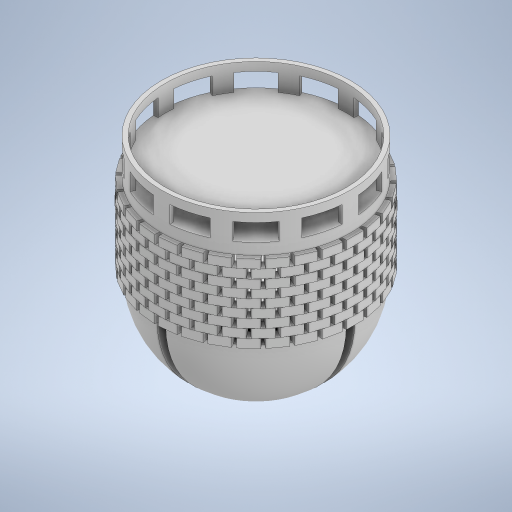
# Autodesk Inventor part: 背部建築 base
Saved by Autodesk Inventor 2024 (Build 280153000, 153)
## iProperties
Created: 2024-05-24
Part Number: 背部建築 base
Material: 一般
Document SubType Name: Modeling
Designer: User
Density: 1 g/cm^3
Appearance: 預設
Author: User
Autodesk Inventor part; units mm, degrees
(part 1 of 2)
ref_plane "YZ Plane" through (0, 0, 0) normal (1, 0, 0) x (0, 1, 0)
ref_plane "XZ Plane" through (0, 0, 0) normal (0, 1, 0) x (-1, 0, 0)
ref_plane "XY Plane" through (0, 0, 0) normal (0, 0, 1) x (1, 0, 0)
sketch "草圖1" plane through (0, 0, 0) normal (0, 1, 0) x (-1, 0, 0)
  circle A0 centre (0, 0) radius 11
  dimension "d0" = 22
  constraints: 1 centre point, 1 coincident
  measures "d0" diameter of A0
extrude "擠出1" add sketch "草圖1" along normal blind 1.3
sketch "草圖2" plane through (0, 1.3, 0) normal (0, 1, 0) x (1, 0, 0)
  line L0 (0, 0) -> (-10.9581, 0.9587)
  circle A0 centre (0, 0) radius 11 projected
  line L1 (0, 0) -> (-10.9581, -0.9587)
  line L2 (-13.6608, 0) -> (-12.5403, 0)
  circle A1 centre (0, 0) radius 10.5
  line L3 (0, 0) -> (-9.9694, -4.6488)
  line L4 (0, 0) -> (-9.0107, -6.3093)
  line L5 (0, 0) -> (-6.3093, -9.0107)
  line L6 (0, 0) -> (-4.6488, -9.9694)
  line L7 (0, 0) -> (-0.9587, -10.9581)
  line L8 (0, 0) -> (0.9587, -10.9581)
  line L9 (0, 0) -> (4.6488, -9.9694)
  line L10 (0, 0) -> (6.3093, -9.0107)
  line L11 (0, 0) -> (9.0107, -6.3093)
  line L12 (0, 0) -> (9.9694, -4.6488)
  line L13 (0, 0) -> (10.9581, -0.9587)
  line L14 (0, 0) -> (10.9581, 0.9587)
  line L15 (0, 0) -> (9.9694, 4.6488)
  line L16 (0, 0) -> (9.0107, 6.3093)
  line L17 (0, 0) -> (6.3093, 9.0107)
  line L18 (0, 0) -> (4.6488, 9.9694)
  line L19 (0, 0) -> (0.9587, 10.9581)
  line L20 (0, 0) -> (-0.9587, 10.9581)
  line L21 (0, 0) -> (-4.6488, 9.9694)
  line L22 (0, 0) -> (-6.3093, 9.0107)
  line L23 (0, 0) -> (-9.0107, 6.3093)
  line L24 (0, 0) -> (-9.9694, 4.6488)
  point P0 (9.5162, -4.4375)
  point P1 (8.6011, -6.0226)
  point P2 (10.46, 0.9151)
  point P3 (10.46, -0.9151)
  point P4 (8.6011, 6.0226)
  point P5 (9.5162, 4.4375)
  point P6 (4.4375, 9.5162)
  point P7 (6.0226, 8.6011)
  point P8 (-0.9151, 10.46)
  point P9 (0.9151, 10.46)
  point P10 (-6.0226, 8.6011)
  point P11 (-4.4375, 9.5162)
  point P12 (-9.5162, 4.4375)
  point P13 (-8.6011, 6.0226)
  point P14 (-10.46, -0.9151)
  point P15 (-10.46, 0.9151)
  point P16 (-8.6011, -6.0226)
  point P17 (-9.5162, -4.4375)
  point P18 (-4.4375, -9.5162)
  point P19 (-6.0226, -8.6011)
  point P20 (0.9151, -10.46)
  point P21 (-0.9151, -10.46)
  point P22 (6.0226, -8.6011)
  point P23 (4.4375, -9.5162)
  dimension "d5" = 21
  dimension "d3" = 5
  dimension "d4" = 5
  dimension "d8" = 360
  constraints: 50 end point, 2 horizontal, 1 coincident, 66 other
  measures "d3" angle of L2 L0
  measures "d4" angle of L2 L1
extrude "擠出2" add sketch "草圖2" along normal blind 2 contours A1 L1 A0 L0 | A1 L4 A0 L3 | A1 L6 A0 L5 | A1 L8 A0 L7 | A1 L10 A0 L9 | A1 L12 A0 L11 | A1 L14 A0 L13 | A1 L16 A0 L15 | A1 L18 A0 L17 | A1 L20 A0 L19 | A1 L22 A0 L21 | A1 L24 A0 L23
sketch "草圖3" plane through (0, 3.3, 0) normal (0, 1, 0) x (1, 0, 0)
  circle A0 centre (0, 0) radius 10.5
  circle A1 centre (0, 0) radius 11
  constraints: 2 centre point, 2 coincident
extrude "擠出3" add sketch "草圖3" along normal blind 1
sketch "草圖4" plane through (0, 0, 0) normal (0, -1, 0) x (1, 0, 0)
  circle A0 centre (0, 0) radius 11
  line L0 (-10.5, -1) -> (-11.5, -1)
  line L1 (-11.5, -1) -> (-11.5, 1)
  line L2 (-11.5, 1) -> (-10.5, 1)
  line L3 (-10.5, 1) -> (-10.5, -1)
  line L4 (-10.5, -1) -> (-11.5, 1) construction
  line L5 (-11.5, -1) -> (-10.5, 1) construction
  line L6 (-11.4566, -1.4128) -> (-10.4785, -1.2049)
  line L7 (-11.0408, -3.3691) -> (-11.4566, -1.4128)
  line L8 (-10.0626, -3.1612) -> (-11.0408, -3.3691)
  line L9 (-10.4785, -1.2049) -> (-10.0626, -3.1612)
  line L10 (-10.9125, -3.7639) -> (-9.999, -3.3572)
  line L11 (-10.099, -5.591) -> (-10.9125, -3.7639)
  line L12 (-9.1855, -5.1843) -> (-10.099, -5.591)
  line L13 (-9.999, -3.3572) -> (-9.1855, -5.1843)
  line L14 (-9.8915, -5.9505) -> (-9.0825, -5.3627)
  line L15 (-8.7159, -7.5685) -> (-9.8915, -5.9505)
  line L16 (-7.9069, -6.9808) -> (-8.7159, -7.5685)
  line L17 (-9.0825, -5.3627) -> (-7.9069, -6.9808)
  line L18 (-8.4381, -7.877) -> (-7.769, -7.1339)
  line L19 (-6.9519, -9.2153) -> (-8.4381, -7.877)
  line L20 (-6.2827, -8.4722) -> (-6.9519, -9.2153)
  line L21 (-7.769, -7.1339) -> (-6.2827, -8.4722)
  line L22 (-6.616, -9.4593) -> (-6.116, -8.5933)
  line L23 (-4.884, -10.4593) -> (-6.616, -9.4593)
  line L24 (-4.384, -9.5933) -> (-4.884, -10.4593)
  line L25 (-6.116, -8.5933) -> (-4.384, -9.5933)
  line L26 (-4.5048, -10.6281) -> (-4.1957, -9.6771)
  line L27 (-2.6026, -11.2462) -> (-4.5048, -10.6281)
  line L28 (-2.2936, -10.2951) -> (-2.6026, -11.2462)
  line L29 (-4.1957, -9.6771) -> (-2.2936, -10.2951)
  line L30 (-2.1966, -11.3325) -> (-2.0921, -10.338)
  line L31 (-0.2076, -11.5415) -> (-2.1966, -11.3325)
  line L32 (-0.103, -10.547) -> (-0.2076, -11.5415)
  line L33 (-2.0921, -10.338) -> (-0.103, -10.547)
  line L34 (0.2076, -11.5415) -> (0.103, -10.547)
  line L35 (2.1966, -11.3325) -> (0.2076, -11.5415)
  line L36 (2.0921, -10.338) -> (2.1966, -11.3325)
  line L37 (0.103, -10.547) -> (2.0921, -10.338)
  line L38 (2.6026, -11.2462) -> (2.2936, -10.2951)
  line L39 (4.5048, -10.6281) -> (2.6026, -11.2462)
  line L40 (4.1957, -9.6771) -> (4.5048, -10.6281)
  line L41 (2.2936, -10.2951) -> (4.1957, -9.6771)
  line L42 (4.884, -10.4593) -> (4.384, -9.5933)
  line L43 (6.616, -9.4593) -> (4.884, -10.4593)
  line L44 (6.116, -8.5933) -> (6.616, -9.4593)
  line L45 (4.384, -9.5933) -> (6.116, -8.5933)
  line L46 (6.9519, -9.2153) -> (6.2827, -8.4722)
  line L47 (8.4381, -7.877) -> (6.9519, -9.2153)
  line L48 (7.769, -7.1339) -> (8.4381, -7.877)
  line L49 (6.2827, -8.4722) -> (7.769, -7.1339)
  line L50 (8.7159, -7.5685) -> (7.9069, -6.9808)
  line L51 (9.8915, -5.9505) -> (8.7159, -7.5685)
  line L52 (9.0825, -5.3627) -> (9.8915, -5.9505)
  line L53 (7.9069, -6.9808) -> (9.0825, -5.3627)
  line L54 (10.099, -5.591) -> (9.1855, -5.1843)
  line L55 (10.9125, -3.7639) -> (10.099, -5.591)
  line L56 (9.999, -3.3572) -> (10.9125, -3.7639)
  line L57 (9.1855, -5.1843) -> (9.999, -3.3572)
  line L58 (11.0408, -3.3691) -> (10.0626, -3.1612)
  line L59 (11.4566, -1.4128) -> (11.0408, -3.3691)
  line L60 (10.4785, -1.2049) -> (11.4566, -1.4128)
  line L61 (10.0626, -3.1612) -> (10.4785, -1.2049)
  line L62 (11.5, -1) -> (10.5, -1)
  line L63 (11.5, 1) -> (11.5, -1)
  line L64 (10.5, 1) -> (11.5, 1)
  line L65 (10.5, -1) -> (10.5, 1)
  line L66 (11.4566, 1.4128) -> (10.4785, 1.2049)
  line L67 (11.0408, 3.3691) -> (11.4566, 1.4128)
  line L68 (10.0626, 3.1612) -> (11.0408, 3.3691)
  line L69 (10.4785, 1.2049) -> (10.0626, 3.1612)
  line L70 (10.9125, 3.7639) -> (9.999, 3.3572)
  line L71 (10.099, 5.591) -> (10.9125, 3.7639)
  line L72 (9.1855, 5.1843) -> (10.099, 5.591)
  line L73 (9.999, 3.3572) -> (9.1855, 5.1843)
  line L74 (9.8915, 5.9505) -> (9.0825, 5.3627)
  line L75 (8.7159, 7.5685) -> (9.8915, 5.9505)
  line L76 (7.9069, 6.9808) -> (8.7159, 7.5685)
  line L77 (9.0825, 5.3627) -> (7.9069, 6.9808)
  line L78 (8.4381, 7.877) -> (7.769, 7.1339)
  line L79 (6.9519, 9.2153) -> (8.4381, 7.877)
  line L80 (6.2827, 8.4722) -> (6.9519, 9.2153)
  line L81 (7.769, 7.1339) -> (6.2827, 8.4722)
  line L82 (6.616, 9.4593) -> (6.116, 8.5933)
  line L83 (4.884, 10.4593) -> (6.616, 9.4593)
  line L84 (4.384, 9.5933) -> (4.884, 10.4593)
  line L85 (6.116, 8.5933) -> (4.384, 9.5933)
  line L86 (4.5048, 10.6281) -> (4.1957, 9.6771)
  line L87 (2.6026, 11.2462) -> (4.5048, 10.6281)
  line L88 (2.2936, 10.2951) -> (2.6026, 11.2462)
  line L89 (4.1957, 9.6771) -> (2.2936, 10.2951)
  line L90 (2.1966, 11.3325) -> (2.0921, 10.338)
  line L91 (0.2076, 11.5415) -> (2.1966, 11.3325)
  line L92 (0.103, 10.547) -> (0.2076, 11.5415)
  line L93 (2.0921, 10.338) -> (0.103, 10.547)
  line L94 (-0.2076, 11.5415) -> (-0.103, 10.547)
  line L95 (-2.1966, 11.3325) -> (-0.2076, 11.5415)
  line L96 (-2.0921, 10.338) -> (-2.1966, 11.3325)
  line L97 (-0.103, 10.547) -> (-2.0921, 10.338)
  line L98 (-2.6026, 11.2462) -> (-2.2936, 10.2951)
  line L99 (-4.5048, 10.6281) -> (-2.6026, 11.2462)
  line L100 (-4.1957, 9.6771) -> (-4.5048, 10.6281)
  line L101 (-2.2936, 10.2951) -> (-4.1957, 9.6771)
  line L102 (-4.884, 10.4593) -> (-4.384, 9.5933)
  line L103 (-6.616, 9.4593) -> (-4.884, 10.4593)
  line L104 (-6.116, 8.5933) -> (-6.616, 9.4593)
  line L105 (-4.384, 9.5933) -> (-6.116, 8.5933)
  line L106 (-6.9519, 9.2153) -> (-6.2827, 8.4722)
  line L107 (-8.4381, 7.877) -> (-6.9519, 9.2153)
  line L108 (-7.769, 7.1339) -> (-8.4381, 7.877)
  line L109 (-6.2827, 8.4722) -> (-7.769, 7.1339)
  line L110 (-8.7159, 7.5685) -> (-7.9069, 6.9808)
  line L111 (-9.8915, 5.9505) -> (-8.7159, 7.5685)
  line L112 (-9.0825, 5.3627) -> (-9.8915, 5.9505)
  line L113 (-7.9069, 6.9808) -> (-9.0825, 5.3627)
  line L114 (-10.099, 5.591) -> (-9.1855, 5.1843)
  line L115 (-10.9125, 3.7639) -> (-10.099, 5.591)
  line L116 (-9.999, 3.3572) -> (-10.9125, 3.7639)
  line L117 (-9.1855, 5.1843) -> (-9.999, 3.3572)
  line L118 (-11.0408, 3.3691) -> (-10.0626, 3.1612)
  line L119 (-11.4566, 1.4128) -> (-11.0408, 3.3691)
  line L120 (-10.4785, 1.2049) -> (-11.4566, 1.4128)
  line L121 (-10.0626, 3.1612) -> (-10.4785, 1.2049)
  point P0 (-11, 0)
  dimension "d14" = 1
  dimension "d15" = 2
  dimension "d18" = 360
  constraints: 244 end point, 2 midpoint, 2 parallel, 1 coincident, 1 horizontal, 1 horizontal alignment, 1 perpendicular, 243 other
  measures "d14" distance of L1.end L2.end
  measures "d15" distance of L0.end L1.end
extrude "擠出4" add sketch "草圖4" along normal blind 1 contours A0 L62 L65 L64 | A0 L64 L63 L62 | L66 L69 L68 A0 | A0 L68 L67 L66 | L60 L59 L58 A0 | A0 L58 L61 L60 | L70 L73 L72 A0 | A0 L72 L71 L70 | L56 L55 L54 A0 | A0 L54 L57 L56 | L74 L77 L76 A0 | A0 L76 L75 L74 | L52 L51 L50 A0 | A0 L50 L53 L52 | L78 L81 L80 A0 | A0 L80 L79 L78 | L48 L47 L46 A0 | A0 L46 L49 L48 | L82 L85 L84 A0 | A0 L84 L83 L82 | L44 L43 L42 A0 | A0 L42 L45 L44 | L86 L89 L88 A0 | A0 L88 L87 L86 | L40 L39 L38 A0 | A0 L38 L41 L40 | L90 L93 L92 A0 | A0 L92 L91 L90 | L36 L35 L34 A0 | A0 L34 L37 L36 | L94 L97 L96 A0 | A0 L96 L95 L94 | L32 L31 L30 A0 | A0 L30 L33 L32 | L98 L101 L100 A0 | A0 L100 L99 L98 | L28 L27 L26 A0 | A0 L26 L29 L28 | L102 L105 L104 A0 | A0 L104 L103 L102 | L24 L23 L22 A0 | A0 L22 L25 L24 | L106 L109 L108 A0 | A0 L108 L107 L106 | L20 L19 L18 A0 | A0 L18 L21 L20 | L110 L113 L112 A0 | A0 L112 L111 L110 | L16 L15 L14 A0 | A0 L14 L17 L16 | L114 L117 L116 A0 | A0 L116 L115 L114 | L12 L11 L10 A0 | A0 L10 L13 L12 | L118 L121 L120 A0 | A0 L120 L119 L118 | L8 L7 L6 A0 | A0 L6 L9 L8 | L2 L3 L0 A0 | A0 L0 L1 L2
sketch "草圖5" plane through (0, -1, 0) normal (0, -1, 0) x (1, 0, 0)
  circle A0 centre (0, 0) radius 11
  line L0 (-1, 10.5) -> (1, 10.5)
  line L1 (1, 10.5) -> (1, 11.5)
  line L2 (1, 11.5) -> (-1, 11.5)
  line L3 (-1, 11.5) -> (-1, 10.5)
  line L4 (-1, 10.5) -> (1, 11.5) construction
  line L5 (1, 10.5) -> (-1, 11.5) construction
  line L6 (-1.2049, 10.4785) -> (-1.4128, 11.4566)
  line L7 (-1.4128, 11.4566) -> (-3.3691, 11.0408)
  line L8 (-3.1612, 10.0626) -> (-1.2049, 10.4785)
  line L9 (-3.3691, 11.0408) -> (-3.1612, 10.0626)
  line L10 (-3.3572, 9.999) -> (-3.7639, 10.9125)
  line L11 (-3.7639, 10.9125) -> (-5.591, 10.099)
  line L12 (-5.1843, 9.1855) -> (-3.3572, 9.999)
  line L13 (-5.591, 10.099) -> (-5.1843, 9.1855)
  line L14 (-5.3627, 9.0825) -> (-5.9505, 9.8915)
  line L15 (-5.9505, 9.8915) -> (-7.5685, 8.7159)
  line L16 (-6.9808, 7.9069) -> (-5.3627, 9.0825)
  line L17 (-7.5685, 8.7159) -> (-6.9808, 7.9069)
  line L18 (-7.1339, 7.769) -> (-7.877, 8.4381)
  line L19 (-7.877, 8.4381) -> (-9.2153, 6.9519)
  line L20 (-8.4722, 6.2827) -> (-7.1339, 7.769)
  line L21 (-9.2153, 6.9519) -> (-8.4722, 6.2827)
  line L22 (-8.5933, 6.116) -> (-9.4593, 6.616)
  line L23 (-9.4593, 6.616) -> (-10.4593, 4.884)
  line L24 (-9.5933, 4.384) -> (-8.5933, 6.116)
  line L25 (-10.4593, 4.884) -> (-9.5933, 4.384)
  line L26 (-9.6771, 4.1957) -> (-10.6281, 4.5048)
  line L27 (-10.6281, 4.5048) -> (-11.2462, 2.6026)
  line L28 (-10.2951, 2.2936) -> (-9.6771, 4.1957)
  line L29 (-11.2462, 2.6026) -> (-10.2951, 2.2936)
  line L30 (-10.338, 2.0921) -> (-11.3325, 2.1966)
  line L31 (-11.3325, 2.1966) -> (-11.5415, 0.2076)
  line L32 (-10.547, 0.103) -> (-10.338, 2.0921)
  line L33 (-11.5415, 0.2076) -> (-10.547, 0.103)
  line L34 (-10.547, -0.103) -> (-11.5415, -0.2076)
  line L35 (-11.5415, -0.2076) -> (-11.3325, -2.1966)
  line L36 (-10.338, -2.0921) -> (-10.547, -0.103)
  line L37 (-11.3325, -2.1966) -> (-10.338, -2.0921)
  line L38 (-10.2951, -2.2936) -> (-11.2462, -2.6026)
  line L39 (-11.2462, -2.6026) -> (-10.6281, -4.5048)
  line L40 (-9.6771, -4.1957) -> (-10.2951, -2.2936)
  line L41 (-10.6281, -4.5048) -> (-9.6771, -4.1957)
  line L42 (-9.5933, -4.384) -> (-10.4593, -4.884)
  line L43 (-10.4593, -4.884) -> (-9.4593, -6.616)
  line L44 (-8.5933, -6.116) -> (-9.5933, -4.384)
  line L45 (-9.4593, -6.616) -> (-8.5933, -6.116)
  line L46 (-8.4722, -6.2827) -> (-9.2153, -6.9519)
  line L47 (-9.2153, -6.9519) -> (-7.877, -8.4381)
  line L48 (-7.1339, -7.769) -> (-8.4722, -6.2827)
  line L49 (-7.877, -8.4381) -> (-7.1339, -7.769)
  line L50 (-6.9808, -7.9069) -> (-7.5685, -8.7159)
  line L51 (-7.5685, -8.7159) -> (-5.9505, -9.8915)
  line L52 (-5.3627, -9.0825) -> (-6.9808, -7.9069)
  line L53 (-5.9505, -9.8915) -> (-5.3627, -9.0825)
  line L54 (-5.1843, -9.1855) -> (-5.591, -10.099)
  line L55 (-5.591, -10.099) -> (-3.7639, -10.9125)
  line L56 (-3.3572, -9.999) -> (-5.1843, -9.1855)
  line L57 (-3.7639, -10.9125) -> (-3.3572, -9.999)
  line L58 (-3.1612, -10.0626) -> (-3.3691, -11.0408)
  line L59 (-3.3691, -11.0408) -> (-1.4128, -11.4566)
  line L60 (-1.2049, -10.4785) -> (-3.1612, -10.0626)
  line L61 (-1.4128, -11.4566) -> (-1.2049, -10.4785)
  line L62 (-1, -10.5) -> (-1, -11.5)
  line L63 (-1, -11.5) -> (1, -11.5)
  line L64 (1, -10.5) -> (-1, -10.5)
  line L65 (1, -11.5) -> (1, -10.5)
  line L66 (1.2049, -10.4785) -> (1.4128, -11.4566)
  line L67 (1.4128, -11.4566) -> (3.3691, -11.0408)
  line L68 (3.1612, -10.0626) -> (1.2049, -10.4785)
  line L69 (3.3691, -11.0408) -> (3.1612, -10.0626)
  line L70 (3.3572, -9.999) -> (3.7639, -10.9125)
  line L71 (3.7639, -10.9125) -> (5.591, -10.099)
  line L72 (5.1843, -9.1855) -> (3.3572, -9.999)
  line L73 (5.591, -10.099) -> (5.1843, -9.1855)
  line L74 (5.3627, -9.0825) -> (5.9505, -9.8915)
  line L75 (5.9505, -9.8915) -> (7.5685, -8.7159)
  line L76 (6.9808, -7.9069) -> (5.3627, -9.0825)
  line L77 (7.5685, -8.7159) -> (6.9808, -7.9069)
  line L78 (7.1339, -7.769) -> (7.877, -8.4381)
  line L79 (7.877, -8.4381) -> (9.2153, -6.9519)
  line L80 (8.4722, -6.2827) -> (7.1339, -7.769)
  line L81 (9.2153, -6.9519) -> (8.4722, -6.2827)
  line L82 (8.5933, -6.116) -> (9.4593, -6.616)
  line L83 (9.4593, -6.616) -> (10.4593, -4.884)
  line L84 (9.5933, -4.384) -> (8.5933, -6.116)
  line L85 (10.4593, -4.884) -> (9.5933, -4.384)
  line L86 (9.6771, -4.1957) -> (10.6281, -4.5048)
  line L87 (10.6281, -4.5048) -> (11.2462, -2.6026)
  line L88 (10.2951, -2.2936) -> (9.6771, -4.1957)
  line L89 (11.2462, -2.6026) -> (10.2951, -2.2936)
  line L90 (10.338, -2.0921) -> (11.3325, -2.1966)
  line L91 (11.3325, -2.1966) -> (11.5415, -0.2076)
  line L92 (10.547, -0.103) -> (10.338, -2.0921)
  line L93 (11.5415, -0.2076) -> (10.547, -0.103)
  line L94 (10.547, 0.103) -> (11.5415, 0.2076)
  line L95 (11.5415, 0.2076) -> (11.3325, 2.1966)
  line L96 (10.338, 2.0921) -> (10.547, 0.103)
  line L97 (11.3325, 2.1966) -> (10.338, 2.0921)
  line L98 (10.2951, 2.2936) -> (11.2462, 2.6026)
  line L99 (11.2462, 2.6026) -> (10.6281, 4.5048)
  line L100 (9.6771, 4.1957) -> (10.2951, 2.2936)
  line L101 (10.6281, 4.5048) -> (9.6771, 4.1957)
  line L102 (9.5933, 4.384) -> (10.4593, 4.884)
  line L103 (10.4593, 4.884) -> (9.4593, 6.616)
  line L104 (8.5933, 6.116) -> (9.5933, 4.384)
  line L105 (9.4593, 6.616) -> (8.5933, 6.116)
  line L106 (8.4722, 6.2827) -> (9.2153, 6.9519)
  line L107 (9.2153, 6.9519) -> (7.877, 8.4381)
  line L108 (7.1339, 7.769) -> (8.4722, 6.2827)
  line L109 (7.877, 8.4381) -> (7.1339, 7.769)
  line L110 (6.9808, 7.9069) -> (7.5685, 8.7159)
  line L111 (7.5685, 8.7159) -> (5.9505, 9.8915)
  line L112 (5.3627, 9.0825) -> (6.9808, 7.9069)
  line L113 (5.9505, 9.8915) -> (5.3627, 9.0825)
  line L114 (5.1843, 9.1855) -> (5.591, 10.099)
  line L115 (5.591, 10.099) -> (3.7639, 10.9125)
  line L116 (3.3572, 9.999) -> (5.1843, 9.1855)
  line L117 (3.7639, 10.9125) -> (3.3572, 9.999)
  line L118 (3.1612, 10.0626) -> (3.3691, 11.0408)
  line L119 (3.3691, 11.0408) -> (1.4128, 11.4566)
  line L120 (1.2049, 10.4785) -> (3.1612, 10.0626)
  line L121 (1.4128, 11.4566) -> (1.2049, 10.4785)
  point P0 (0, 11)
  dimension "d22" = 2
  dimension "d23" = 1
  dimension "d26" = 360
  constraints: 244 end point, 2 midpoint, 2 parallel, 1 coincident, 1 horizontal, 1 perpendicular, 1 vertical alignment, 243 other
  measures "d22" distance of L2.end L1.end
  measures "d23" distance of L1.end L0.end
extrude "擠出5" add sketch "草圖5" along normal blind 1 contours L94 L96 L97 A0 | A0 L97 L95 L94 | L93 L91 L90 A0 | A0 L90 L92 L93 | L98 L100 L101 A0 | A0 L101 L99 L98 | L89 L87 L86 A0 | A0 L86 L88 L89 | L102 L104 L105 A0 | A0 L105 L103 L102 | L85 L83 L82 A0 | A0 L82 L84 L85 | L106 L108 L109 A0 | A0 L109 L107 L106 | L81 L79 L78 A0 | A0 L78 L80 L81 | L110 L112 L113 A0 | A0 L113 L111 L110 | L77 L75 L74 A0 | A0 L74 L76 L77 | L114 L116 L117 A0 | A0 L117 L115 L114 | L73 L71 L70 A0 | A0 L70 L72 L73 | L118 L120 L121 A0 | A0 L121 L119 L118 | L69 L67 L66 A0 | A0 L66 L68 L69 | L1 L0 L3 A0 | A0 L3 L2 L1 | L65 L63 L62 A0 | A0 L62 L64 L65 | L6 L8 L9 A0 | A0 L9 L7 L6 | L61 L59 L58 A0 | A0 L58 L60 L61 | L10 L12 L13 A0 | A0 L13 L11 L10 | L57 L55 L54 A0 | A0 L54 L56 L57 | L14 L16 L17 A0 | A0 L17 L15 L14 | L53 L51 L50 A0 | A0 L50 L52 L53 | L18 L20 L21 A0 | A0 L21 L19 L18 | L49 L47 L46 A0 | A0 L46 L48 L49 | L22 L24 L25 A0 | A0 L25 L23 L22 | L45 L43 L42 A0 | A0 L42 L44 L45 | L26 L28 L29 A0 | A0 L29 L27 L26 | L41 L39 L38 A0 | A0 L38 L40 L41 | L30 L32 L33 A0 | A0 L33 L31 L30 | L37 L35 L34 A0 | A0 L34 L36 L37
sketch "草圖6" plane through (0, -2, 0) normal (0, -1, 0) x (1, 0, 0)
  circle A0 centre (0, 0) radius 11.0454
  line L0 (-11.5454, -1) -> (-10.5454, -1)
  line L1 (-10.5454, -1) -> (-10.5454, 1)
  line L2 (-10.5454, 1) -> (-11.5454, 1)
  line L3 (-11.5454, 1) -> (-11.5454, -1)
  line L4 (-11.5454, -1) -> (-10.5454, 1) construction
  line L5 (-10.5454, -1) -> (-11.5454, 1) construction
  line L6 (-10.5228, -1.2144) -> (-11.501, -1.4223)
  line L7 (-10.107, -3.1707) -> (-10.5228, -1.2144)
  line L8 (-11.501, -1.4223) -> (-11.0852, -3.3786)
  line L9 (-11.0852, -3.3786) -> (-10.107, -3.1707)
  line L10 (-10.0404, -3.3756) -> (-10.9539, -3.7824)
  line L11 (-9.2269, -5.2027) -> (-10.0404, -3.3756)
  line L12 (-10.9539, -3.7824) -> (-10.1405, -5.6095)
  line L13 (-10.1405, -5.6095) -> (-9.2269, -5.2027)
  line L14 (-9.1192, -5.3894) -> (-9.9282, -5.9772)
  line L15 (-7.9436, -7.0074) -> (-9.1192, -5.3894)
  line L16 (-9.9282, -5.9772) -> (-8.7526, -7.5952)
  line L17 (-8.7526, -7.5952) -> (-7.9436, -7.0074)
  line L18 (-7.7994, -7.1676) -> (-8.4685, -7.9107)
  line L19 (-6.3131, -8.5059) -> (-7.7994, -7.1676)
  line L20 (-8.4685, -7.9107) -> (-6.9822, -9.249)
  line L21 (-6.9822, -9.249) -> (-6.3131, -8.5059)
  line L22 (-6.1387, -8.6326) -> (-6.6387, -9.4986)
  line L23 (-4.4067, -9.6326) -> (-6.1387, -8.6326)
  line L24 (-6.6387, -9.4986) -> (-4.9067, -10.4986)
  line L25 (-4.9067, -10.4986) -> (-4.4067, -9.6326)
  line L26 (-4.2098, -9.7202) -> (-4.5188, -10.6713)
  line L27 (-2.3076, -10.3383) -> (-4.2098, -9.7202)
  line L28 (-4.5188, -10.6713) -> (-2.6167, -11.2893)
  line L29 (-2.6167, -11.2893) -> (-2.3076, -10.3383)
  line L30 (-2.0968, -10.3831) -> (-2.2013, -11.3776)
  line L31 (-0.1078, -10.5921) -> (-2.0968, -10.3831)
  line L32 (-2.2013, -11.3776) -> (-0.2123, -11.5866)
  line L33 (-0.2123, -11.5866) -> (-0.1078, -10.5921)
  line L34 (0.1078, -10.5921) -> (0.2123, -11.5866)
  line L35 (2.0968, -10.3831) -> (0.1078, -10.5921)
  line L36 (0.2123, -11.5866) -> (2.2013, -11.3776)
  line L37 (2.2013, -11.3776) -> (2.0968, -10.3831)
  line L38 (2.3076, -10.3383) -> (2.6167, -11.2893)
  line L39 (4.2098, -9.7202) -> (2.3076, -10.3383)
  line L40 (2.6167, -11.2893) -> (4.5188, -10.6713)
  line L41 (4.5188, -10.6713) -> (4.2098, -9.7202)
  line L42 (4.4067, -9.6326) -> (4.9067, -10.4986)
  line L43 (6.1387, -8.6326) -> (4.4067, -9.6326)
  line L44 (4.9067, -10.4986) -> (6.6387, -9.4986)
  line L45 (6.6387, -9.4986) -> (6.1387, -8.6326)
  line L46 (6.3131, -8.5059) -> (6.9822, -9.249)
  line L47 (7.7994, -7.1676) -> (6.3131, -8.5059)
  line L48 (6.9822, -9.249) -> (8.4685, -7.9107)
  line L49 (8.4685, -7.9107) -> (7.7994, -7.1676)
  line L50 (7.9436, -7.0074) -> (8.7526, -7.5952)
  line L51 (9.1192, -5.3894) -> (7.9436, -7.0074)
  line L52 (8.7526, -7.5952) -> (9.9282, -5.9772)
  line L53 (9.9282, -5.9772) -> (9.1192, -5.3894)
  line L54 (9.2269, -5.2027) -> (10.1405, -5.6095)
  line L55 (10.0404, -3.3756) -> (9.2269, -5.2027)
  line L56 (10.1405, -5.6095) -> (10.9539, -3.7824)
  line L57 (10.9539, -3.7824) -> (10.0404, -3.3756)
  line L58 (10.107, -3.1707) -> (11.0852, -3.3786)
  line L59 (10.5228, -1.2144) -> (10.107, -3.1707)
  line L60 (11.0852, -3.3786) -> (11.501, -1.4223)
  line L61 (11.501, -1.4223) -> (10.5228, -1.2144)
  line L62 (10.5454, -1) -> (11.5454, -1)
  line L63 (10.5454, 1) -> (10.5454, -1)
  line L64 (11.5454, -1) -> (11.5454, 1)
  line L65 (11.5454, 1) -> (10.5454, 1)
  line L66 (10.5228, 1.2144) -> (11.501, 1.4223)
  line L67 (10.107, 3.1707) -> (10.5228, 1.2144)
  line L68 (11.501, 1.4223) -> (11.0852, 3.3786)
  line L69 (11.0852, 3.3786) -> (10.107, 3.1707)
  line L70 (10.0404, 3.3756) -> (10.9539, 3.7824)
  line L71 (9.2269, 5.2027) -> (10.0404, 3.3756)
  line L72 (10.9539, 3.7824) -> (10.1405, 5.6095)
  line L73 (10.1405, 5.6095) -> (9.2269, 5.2027)
  line L74 (9.1192, 5.3894) -> (9.9282, 5.9772)
  line L75 (7.9436, 7.0074) -> (9.1192, 5.3894)
  line L76 (9.9282, 5.9772) -> (8.7526, 7.5952)
  line L77 (8.7526, 7.5952) -> (7.9436, 7.0074)
  line L78 (7.7994, 7.1676) -> (8.4685, 7.9107)
  line L79 (6.3131, 8.5059) -> (7.7994, 7.1676)
  line L80 (8.4685, 7.9107) -> (6.9822, 9.249)
  line L81 (6.9822, 9.249) -> (6.3131, 8.5059)
  line L82 (6.1387, 8.6326) -> (6.6387, 9.4986)
  line L83 (4.4067, 9.6326) -> (6.1387, 8.6326)
  line L84 (6.6387, 9.4986) -> (4.9067, 10.4986)
  line L85 (4.9067, 10.4986) -> (4.4067, 9.6326)
  line L86 (4.2098, 9.7202) -> (4.5188, 10.6713)
  line L87 (2.3076, 10.3383) -> (4.2098, 9.7202)
  line L88 (4.5188, 10.6713) -> (2.6167, 11.2893)
  line L89 (2.6167, 11.2893) -> (2.3076, 10.3383)
  line L90 (2.0968, 10.3831) -> (2.2013, 11.3776)
  line L91 (0.1078, 10.5921) -> (2.0968, 10.3831)
  line L92 (2.2013, 11.3776) -> (0.2123, 11.5866)
  line L93 (0.2123, 11.5866) -> (0.1078, 10.5921)
  line L94 (-0.1078, 10.5921) -> (-0.2123, 11.5866)
  line L95 (-2.0968, 10.3831) -> (-0.1078, 10.5921)
  line L96 (-0.2123, 11.5866) -> (-2.2013, 11.3776)
  line L97 (-2.2013, 11.3776) -> (-2.0968, 10.3831)
  line L98 (-2.3076, 10.3383) -> (-2.6167, 11.2893)
  line L99 (-4.2098, 9.7202) -> (-2.3076, 10.3383)
  line L100 (-2.6167, 11.2893) -> (-4.5188, 10.6713)
  line L101 (-4.5188, 10.6713) -> (-4.2098, 9.7202)
  line L102 (-4.4067, 9.6326) -> (-4.9067, 10.4986)
  line L103 (-6.1387, 8.6326) -> (-4.4067, 9.6326)
  line L104 (-4.9067, 10.4986) -> (-6.6387, 9.4986)
  line L105 (-6.6387, 9.4986) -> (-6.1387, 8.6326)
  line L106 (-6.3131, 8.5059) -> (-6.9822, 9.249)
  line L107 (-7.7994, 7.1676) -> (-6.3131, 8.5059)
  line L108 (-6.9822, 9.249) -> (-8.4685, 7.9107)
  line L109 (-8.4685, 7.9107) -> (-7.7994, 7.1676)
  line L110 (-7.9436, 7.0074) -> (-8.7526, 7.5952)
  line L111 (-9.1192, 5.3894) -> (-7.9436, 7.0074)
  line L112 (-8.7526, 7.5952) -> (-9.9282, 5.9772)
  line L113 (-9.9282, 5.9772) -> (-9.1192, 5.3894)
  line L114 (-9.2269, 5.2027) -> (-10.1405, 5.6095)
  line L115 (-10.0404, 3.3756) -> (-9.2269, 5.2027)
  line L116 (-10.1405, 5.6095) -> (-10.9539, 3.7824)
  line L117 (-10.9539, 3.7824) -> (-10.0404, 3.3756)
  line L118 (-10.107, 3.1707) -> (-11.0852, 3.3786)
  line L119 (-10.5228, 1.2144) -> (-10.107, 3.1707)
  line L120 (-11.0852, 3.3786) -> (-11.501, 1.4223)
  line L121 (-11.501, 1.4223) -> (-10.5228, 1.2144)
  point P0 (-11.0454, 0)
  dimension "d30" = 1
  dimension "d31" = 2
  dimension "d34" = 360
  constraints: 244 end point, 2 midpoint, 2 parallel, 1 coincident, 1 horizontal, 1 horizontal alignment, 1 perpendicular, 243 other
  measures "d30" distance of L2.end L1.end
  measures "d31" distance of L1.end L0.end
extrude "擠出6" add sketch "草圖6" along normal blind 1 contours A0 L62 L63 L65 | A0 L65 L64 L62 | L66 L67 L69 A0 | A0 L69 L68 L66 | L61 L60 L58 A0 | A0 L58 L59 L61 | L70 L71 L73 A0 | A0 L73 L72 L70 | L57 L56 L54 A0 | A0 L54 L55 L57 | L74 L75 L77 A0 | A0 L77 L76 L74 | L53 L52 L50 A0 | A0 L50 L51 L53 | L78 L79 L81 A0 | A0 L81 L80 L78 | L49 L48 L46 A0 | A0 L46 L47 L49 | L82 L83 L85 A0 | A0 L85 L84 L82 | L45 L44 L42 A0 | A0 L42 L43 L45 | L86 L87 L89 A0 | A0 L89 L88 L86 | L41 L40 L38 A0 | A0 L38 L39 L41 | L90 L91 L93 A0 | A0 L93 L92 L90 | L37 L36 L34 A0 | A0 L34 L35 L37 | L94 L95 L97 A0 | A0 L97 L96 L94 | L33 L32 L30 A0 | A0 L30 L31 L33 | L98 L99 L101 A0 | A0 L101 L100 L98 | L29 L28 L26 A0 | A0 L26 L27 L29 | L102 L103 L105 A0 | A0 L105 L104 L102 | L25 L24 L22 A0 | A0 L22 L23 L25 | L106 L107 L109 A0 | A0 L109 L108 L106 | L21 L20 L18 A0 | A0 L18 L19 L21 | L110 L111 L113 A0 | A0 L113 L112 L110 | L17 L16 L14 A0 | A0 L14 L15 L17 | L114 L115 L117 A0 | A0 L117 L116 L114 | L13 L12 L10 A0 | A0 L10 L11 L13 | L118 L119 L121 A0 | A0 L121 L120 L118 | L9 L8 L6 A0 | A0 L6 L7 L9 | L2 L1 L0 A0 | A0 L0 L3 L2
sketch "草圖7" plane through (0, -3, 0) normal (0, -1, 0) x (1, 0, 0)
  circle A0 centre (0, 0) radius 11
  line L0 (-1, 10.5) -> (1, 10.5)
  line L1 (1, 10.5) -> (1, 11.5)
  line L2 (1, 11.5) -> (-1, 11.5)
  line L3 (-1, 11.5) -> (-1, 10.5)
  line L4 (-1, 10.5) -> (1, 11.5) construction
  line L5 (1, 10.5) -> (-1, 11.5) construction
  line L6 (-1.2049, 10.4785) -> (-1.4128, 11.4566)
  line L7 (-1.4128, 11.4566) -> (-3.3691, 11.0408)
  line L8 (-3.1612, 10.0626) -> (-1.2049, 10.4785)
  line L9 (-3.3691, 11.0408) -> (-3.1612, 10.0626)
  line L10 (-3.3572, 9.999) -> (-3.7639, 10.9125)
  line L11 (-3.7639, 10.9125) -> (-5.591, 10.099)
  line L12 (-5.1843, 9.1855) -> (-3.3572, 9.999)
  line L13 (-5.591, 10.099) -> (-5.1843, 9.1855)
  line L14 (-5.3627, 9.0825) -> (-5.9505, 9.8915)
  line L15 (-5.9505, 9.8915) -> (-7.5685, 8.7159)
  line L16 (-6.9808, 7.9069) -> (-5.3627, 9.0825)
  line L17 (-7.5685, 8.7159) -> (-6.9808, 7.9069)
  line L18 (-7.1339, 7.769) -> (-7.877, 8.4381)
  line L19 (-7.877, 8.4381) -> (-9.2153, 6.9519)
  line L20 (-8.4722, 6.2827) -> (-7.1339, 7.769)
  line L21 (-9.2153, 6.9519) -> (-8.4722, 6.2827)
  line L22 (-8.5933, 6.116) -> (-9.4593, 6.616)
  line L23 (-9.4593, 6.616) -> (-10.4593, 4.884)
  line L24 (-9.5933, 4.384) -> (-8.5933, 6.116)
  line L25 (-10.4593, 4.884) -> (-9.5933, 4.384)
  line L26 (-9.6771, 4.1957) -> (-10.6281, 4.5048)
  line L27 (-10.6281, 4.5048) -> (-11.2462, 2.6026)
  line L28 (-10.2951, 2.2936) -> (-9.6771, 4.1957)
  line L29 (-11.2462, 2.6026) -> (-10.2951, 2.2936)
  line L30 (-10.338, 2.0921) -> (-11.3325, 2.1966)
  line L31 (-11.3325, 2.1966) -> (-11.5415, 0.2076)
  line L32 (-10.547, 0.103) -> (-10.338, 2.0921)
  line L33 (-11.5415, 0.2076) -> (-10.547, 0.103)
  line L34 (-10.547, -0.103) -> (-11.5415, -0.2076)
  line L35 (-11.5415, -0.2076) -> (-11.3325, -2.1966)
  line L36 (-10.338, -2.0921) -> (-10.547, -0.103)
  line L37 (-11.3325, -2.1966) -> (-10.338, -2.0921)
  line L38 (-10.2951, -2.2936) -> (-11.2462, -2.6026)
  line L39 (-11.2462, -2.6026) -> (-10.6281, -4.5048)
  line L40 (-9.6771, -4.1957) -> (-10.2951, -2.2936)
  line L41 (-10.6281, -4.5048) -> (-9.6771, -4.1957)
  line L42 (-9.5933, -4.384) -> (-10.4593, -4.884)
  line L43 (-10.4593, -4.884) -> (-9.4593, -6.616)
  line L44 (-8.5933, -6.116) -> (-9.5933, -4.384)
  line L45 (-9.4593, -6.616) -> (-8.5933, -6.116)
  line L46 (-8.4722, -6.2827) -> (-9.2153, -6.9519)
  line L47 (-9.2153, -6.9519) -> (-7.877, -8.4381)
  line L48 (-7.1339, -7.769) -> (-8.4722, -6.2827)
  line L49 (-7.877, -8.4381) -> (-7.1339, -7.769)
  line L50 (-6.9808, -7.9069) -> (-7.5685, -8.7159)
  line L51 (-7.5685, -8.7159) -> (-5.9505, -9.8915)
  line L52 (-5.3627, -9.0825) -> (-6.9808, -7.9069)
  line L53 (-5.9505, -9.8915) -> (-5.3627, -9.0825)
  line L54 (-5.1843, -9.1855) -> (-5.591, -10.099)
  line L55 (-5.591, -10.099) -> (-3.7639, -10.9125)
  line L56 (-3.3572, -9.999) -> (-5.1843, -9.1855)
  line L57 (-3.7639, -10.9125) -> (-3.3572, -9.999)
  line L58 (-3.1612, -10.0626) -> (-3.3691, -11.0408)
  line L59 (-3.3691, -11.0408) -> (-1.4128, -11.4566)
  line L60 (-1.2049, -10.4785) -> (-3.1612, -10.0626)
  line L61 (-1.4128, -11.4566) -> (-1.2049, -10.4785)
  line L62 (-1, -10.5) -> (-1, -11.5)
  line L63 (-1, -11.5) -> (1, -11.5)
  line L64 (1, -10.5) -> (-1, -10.5)
  line L65 (1, -11.5) -> (1, -10.5)
  line L66 (1.2049, -10.4785) -> (1.4128, -11.4566)
  line L67 (1.4128, -11.4566) -> (3.3691, -11.0408)
  line L68 (3.1612, -10.0626) -> (1.2049, -10.4785)
  line L69 (3.3691, -11.0408) -> (3.1612, -10.0626)
  line L70 (3.3572, -9.999) -> (3.7639, -10.9125)
  line L71 (3.7639, -10.9125) -> (5.591, -10.099)
  line L72 (5.1843, -9.1855) -> (3.3572, -9.999)
  line L73 (5.591, -10.099) -> (5.1843, -9.1855)
  line L74 (5.3627, -9.0825) -> (5.9505, -9.8915)
  line L75 (5.9505, -9.8915) -> (7.5685, -8.7159)
  line L76 (6.9808, -7.9069) -> (5.3627, -9.0825)
  line L77 (7.5685, -8.7159) -> (6.9808, -7.9069)
  line L78 (7.1339, -7.769) -> (7.877, -8.4381)
  line L79 (7.877, -8.4381) -> (9.2153, -6.9519)
  line L80 (8.4722, -6.2827) -> (7.1339, -7.769)
  line L81 (9.2153, -6.9519) -> (8.4722, -6.2827)
  line L82 (8.5933, -6.116) -> (9.4593, -6.616)
  line L83 (9.4593, -6.616) -> (10.4593, -4.884)
  line L84 (9.5933, -4.384) -> (8.5933, -6.116)
  line L85 (10.4593, -4.884) -> (9.5933, -4.384)
  line L86 (9.6771, -4.1957) -> (10.6281, -4.5048)
  line L87 (10.6281, -4.5048) -> (11.2462, -2.6026)
  line L88 (10.2951, -2.2936) -> (9.6771, -4.1957)
  line L89 (11.2462, -2.6026) -> (10.2951, -2.2936)
  line L90 (10.338, -2.0921) -> (11.3325, -2.1966)
  line L91 (11.3325, -2.1966) -> (11.5415, -0.2076)
  line L92 (10.547, -0.103) -> (10.338, -2.0921)
  line L93 (11.5415, -0.2076) -> (10.547, -0.103)
  line L94 (10.547, 0.103) -> (11.5415, 0.2076)
  line L95 (11.5415, 0.2076) -> (11.3325, 2.1966)
  line L96 (10.338, 2.0921) -> (10.547, 0.103)
  line L97 (11.3325, 2.1966) -> (10.338, 2.0921)
  line L98 (10.2951, 2.2936) -> (11.2462, 2.6026)
  line L99 (11.2462, 2.6026) -> (10.6281, 4.5048)
  line L100 (9.6771, 4.1957) -> (10.2951, 2.2936)
  line L101 (10.6281, 4.5048) -> (9.6771, 4.1957)
  line L102 (9.5933, 4.384) -> (10.4593, 4.884)
  line L103 (10.4593, 4.884) -> (9.4593, 6.616)
  line L104 (8.5933, 6.116) -> (9.5933, 4.384)
  line L105 (9.4593, 6.616) -> (8.5933, 6.116)
  line L106 (8.4722, 6.2827) -> (9.2153, 6.9519)
  line L107 (9.2153, 6.9519) -> (7.877, 8.4381)
  line L108 (7.1339, 7.769) -> (8.4722, 6.2827)
  line L109 (7.877, 8.4381) -> (7.1339, 7.769)
  line L110 (6.9808, 7.9069) -> (7.5685, 8.7159)
  line L111 (7.5685, 8.7159) -> (5.9505, 9.8915)
  line L112 (5.3627, 9.0825) -> (6.9808, 7.9069)
  line L113 (5.9505, 9.8915) -> (5.3627, 9.0825)
  line L114 (5.1843, 9.1855) -> (5.591, 10.099)
  line L115 (5.591, 10.099) -> (3.7639, 10.9125)
  line L116 (3.3572, 9.999) -> (5.1843, 9.1855)
  line L117 (3.7639, 10.9125) -> (3.3572, 9.999)
  line L118 (3.1612, 10.0626) -> (3.3691, 11.0408)
  line L119 (3.3691, 11.0408) -> (1.4128, 11.4566)
  line L120 (1.2049, 10.4785) -> (3.1612, 10.0626)
  line L121 (1.4128, 11.4566) -> (1.2049, 10.4785)
  point P0 (0, 11)
  dimension "d38" = 22
  dimension "d39" = 2
  dimension "d40" = 1
  dimension "d43" = 360
  constraints: 244 end point, 2 midpoint, 2 parallel, 1 coincident, 1 horizontal, 1 perpendicular, 1 vertical alignment, 243 other
  measures "d39" distance of L2.end L1.end
  measures "d40" distance of L1.end L0.end
extrude "擠出7" add sketch "草圖7" along normal blind 1 contours L94 L96 L97 A0 | A0 L97 L95 L94 | L93 L91 L90 A0 | A0 L90 L92 L93 | L98 L100 L101 A0 | A0 L101 L99 L98 | L89 L87 L86 A0 | A0 L86 L88 L89 | L102 L104 L105 A0 | A0 L105 L103 L102 | L85 L83 L82 A0 | A0 L82 L84 L85 | L106 L108 L109 A0 | A0 L109 L107 L106 | L81 L79 L78 A0 | A0 L78 L80 L81 | L110 L112 L113 A0 | A0 L113 L111 L110 | L77 L75 L74 A0 | A0 L74 L76 L77 | L114 L116 L117 A0 | A0 L117 L115 L114 | L73 L71 L70 A0 | A0 L70 L72 L73 | L118 L120 L121 A0 | A0 L121 L119 L118 | L69 L67 L66 A0 | A0 L66 L68 L69 | L1 L0 L3 A0 | A0 L3 L2 L1 | L65 L63 L62 A0 | A0 L62 L64 L65 | L6 L8 L9 A0 | A0 L9 L7 L6 | L61 L59 L58 A0 | A0 L58 L60 L61 | L10 L12 L13 A0 | A0 L13 L11 L10 | L57 L55 L54 A0 | A0 L54 L56 L57 | L14 L16 L17 A0 | A0 L17 L15 L14 | L53 L51 L50 A0 | A0 L50 L52 L53 | L18 L20 L21 A0 | A0 L21 L19 L18 | L49 L47 L46 A0 | A0 L46 L48 L49 | L22 L24 L25 A0 | A0 L25 L23 L22 | L45 L43 L42 A0 | A0 L42 L44 L45 | L26 L28 L29 A0 | A0 L29 L27 L26 | L41 L39 L38 A0 | A0 L38 L40 L41 | L30 L32 L33 A0 | A0 L33 L31 L30 | L37 L35 L34 A0 | A0 L34 L36 L37
sketch "草圖8" plane through (0, -4, 0) normal (0, -1, 0) x (1, 0, 0)
  circle A0 centre (0, 0) radius 11
  line L0 (-11.5, -1) -> (-10.5, -1)
  line L1 (-10.5, -1) -> (-10.5, 1)
  line L2 (-10.5, 1) -> (-11.5, 1)
  line L3 (-11.5, 1) -> (-11.5, -1)
  line L4 (-11.5, -1) -> (-10.5, 1) construction
  line L5 (-10.5, -1) -> (-11.5, 1) construction
  line L6 (-10.4785, -1.2049) -> (-11.4566, -1.4128)
  line L7 (-10.0626, -3.1612) -> (-10.4785, -1.2049)
  line L8 (-11.4566, -1.4128) -> (-11.0408, -3.3691)
  line L9 (-11.0408, -3.3691) -> (-10.0626, -3.1612)
  line L10 (-9.999, -3.3572) -> (-10.9125, -3.7639)
  line L11 (-9.1855, -5.1843) -> (-9.999, -3.3572)
  line L12 (-10.9125, -3.7639) -> (-10.099, -5.591)
  line L13 (-10.099, -5.591) -> (-9.1855, -5.1843)
  line L14 (-9.0825, -5.3627) -> (-9.8915, -5.9505)
  line L15 (-7.9069, -6.9808) -> (-9.0825, -5.3627)
  line L16 (-9.8915, -5.9505) -> (-8.7159, -7.5685)
  line L17 (-8.7159, -7.5685) -> (-7.9069, -6.9808)
  line L18 (-7.769, -7.1339) -> (-8.4381, -7.877)
  line L19 (-6.2827, -8.4722) -> (-7.769, -7.1339)
  line L20 (-8.4381, -7.877) -> (-6.9519, -9.2153)
  line L21 (-6.9519, -9.2153) -> (-6.2827, -8.4722)
  line L22 (-6.116, -8.5933) -> (-6.616, -9.4593)
  line L23 (-4.384, -9.5933) -> (-6.116, -8.5933)
  line L24 (-6.616, -9.4593) -> (-4.884, -10.4593)
  line L25 (-4.884, -10.4593) -> (-4.384, -9.5933)
  line L26 (-4.1957, -9.6771) -> (-4.5048, -10.6281)
  line L27 (-2.2936, -10.2951) -> (-4.1957, -9.6771)
  line L28 (-4.5048, -10.6281) -> (-2.6026, -11.2462)
  line L29 (-2.6026, -11.2462) -> (-2.2936, -10.2951)
  line L30 (-2.0921, -10.338) -> (-2.1966, -11.3325)
  line L31 (-0.103, -10.547) -> (-2.0921, -10.338)
  line L32 (-2.1966, -11.3325) -> (-0.2076, -11.5415)
  line L33 (-0.2076, -11.5415) -> (-0.103, -10.547)
  line L34 (0.103, -10.547) -> (0.2076, -11.5415)
  line L35 (2.0921, -10.338) -> (0.103, -10.547)
  line L36 (0.2076, -11.5415) -> (2.1966, -11.3325)
  line L37 (2.1966, -11.3325) -> (2.0921, -10.338)
  line L38 (2.2936, -10.2951) -> (2.6026, -11.2462)
  line L39 (4.1957, -9.6771) -> (2.2936, -10.2951)
  line L40 (2.6026, -11.2462) -> (4.5048, -10.6281)
  line L41 (4.5048, -10.6281) -> (4.1957, -9.6771)
  line L42 (4.384, -9.5933) -> (4.884, -10.4593)
  line L43 (6.116, -8.5933) -> (4.384, -9.5933)
  line L44 (4.884, -10.4593) -> (6.616, -9.4593)
  line L45 (6.616, -9.4593) -> (6.116, -8.5933)
  line L46 (6.2827, -8.4722) -> (6.9519, -9.2153)
  line L47 (7.769, -7.1339) -> (6.2827, -8.4722)
  line L48 (6.9519, -9.2153) -> (8.4381, -7.877)
  line L49 (8.4381, -7.877) -> (7.769, -7.1339)
  line L50 (7.9069, -6.9808) -> (8.7159, -7.5685)
  line L51 (9.0825, -5.3627) -> (7.9069, -6.9808)
  line L52 (8.7159, -7.5685) -> (9.8915, -5.9505)
  line L53 (9.8915, -5.9505) -> (9.0825, -5.3627)
  line L54 (9.1855, -5.1843) -> (10.099, -5.591)
  line L55 (9.999, -3.3572) -> (9.1855, -5.1843)
  line L56 (10.099, -5.591) -> (10.9125, -3.7639)
  line L57 (10.9125, -3.7639) -> (9.999, -3.3572)
  line L58 (10.0626, -3.1612) -> (11.0408, -3.3691)
  line L59 (10.4785, -1.2049) -> (10.0626, -3.1612)
  line L60 (11.0408, -3.3691) -> (11.4566, -1.4128)
  line L61 (11.4566, -1.4128) -> (10.4785, -1.2049)
  line L62 (10.5, -1) -> (11.5, -1)
  line L63 (10.5, 1) -> (10.5, -1)
  line L64 (11.5, -1) -> (11.5, 1)
  line L65 (11.5, 1) -> (10.5, 1)
  line L66 (10.4785, 1.2049) -> (11.4566, 1.4128)
  line L67 (10.0626, 3.1612) -> (10.4785, 1.2049)
  line L68 (11.4566, 1.4128) -> (11.0408, 3.3691)
  line L69 (11.0408, 3.3691) -> (10.0626, 3.1612)
  line L70 (9.999, 3.3572) -> (10.9125, 3.7639)
  line L71 (9.1855, 5.1843) -> (9.999, 3.3572)
  line L72 (10.9125, 3.7639) -> (10.099, 5.591)
  line L73 (10.099, 5.591) -> (9.1855, 5.1843)
  line L74 (9.0825, 5.3627) -> (9.8915, 5.9505)
  line L75 (7.9069, 6.9808) -> (9.0825, 5.3627)
  line L76 (9.8915, 5.9505) -> (8.7159, 7.5685)
  line L77 (8.7159, 7.5685) -> (7.9069, 6.9808)
  line L78 (7.769, 7.1339) -> (8.4381, 7.877)
  line L79 (6.2827, 8.4722) -> (7.769, 7.1339)
  line L80 (8.4381, 7.877) -> (6.9519, 9.2153)
  line L81 (6.9519, 9.2153) -> (6.2827, 8.4722)
  line L82 (6.116, 8.5933) -> (6.616, 9.4593)
  line L83 (4.384, 9.5933) -> (6.116, 8.5933)
  line L84 (6.616, 9.4593) -> (4.884, 10.4593)
  line L85 (4.884, 10.4593) -> (4.384, 9.5933)
  line L86 (4.1957, 9.6771) -> (4.5048, 10.6281)
  line L87 (2.2936, 10.2951) -> (4.1957, 9.6771)
  line L88 (4.5048, 10.6281) -> (2.6026, 11.2462)
  line L89 (2.6026, 11.2462) -> (2.2936, 10.2951)
  line L90 (2.0921, 10.338) -> (2.1966, 11.3325)
  line L91 (0.103, 10.547) -> (2.0921, 10.338)
  line L92 (2.1966, 11.3325) -> (0.2076, 11.5415)
  line L93 (0.2076, 11.5415) -> (0.103, 10.547)
  line L94 (-0.103, 10.547) -> (-0.2076, 11.5415)
  line L95 (-2.0921, 10.338) -> (-0.103, 10.547)
  line L96 (-0.2076, 11.5415) -> (-2.1966, 11.3325)
  line L97 (-2.1966, 11.3325) -> (-2.0921, 10.338)
  line L98 (-2.2936, 10.2951) -> (-2.6026, 11.2462)
  line L99 (-4.1957, 9.6771) -> (-2.2936, 10.2951)
  line L100 (-2.6026, 11.2462) -> (-4.5048, 10.6281)
  line L101 (-4.5048, 10.6281) -> (-4.1957, 9.6771)
  line L102 (-4.384, 9.5933) -> (-4.884, 10.4593)
  line L103 (-6.116, 8.5933) -> (-4.384, 9.5933)
  line L104 (-4.884, 10.4593) -> (-6.616, 9.4593)
  line L105 (-6.616, 9.4593) -> (-6.116, 8.5933)
  line L106 (-6.2827, 8.4722) -> (-6.9519, 9.2153)
  line L107 (-7.769, 7.1339) -> (-6.2827, 8.4722)
  line L108 (-6.9519, 9.2153) -> (-8.4381, 7.877)
  line L109 (-8.4381, 7.877) -> (-7.769, 7.1339)
  line L110 (-7.9069, 6.9808) -> (-8.7159, 7.5685)
  line L111 (-9.0825, 5.3627) -> (-7.9069, 6.9808)
  line L112 (-8.7159, 7.5685) -> (-9.8915, 5.9505)
  line L113 (-9.8915, 5.9505) -> (-9.0825, 5.3627)
  line L114 (-9.1855, 5.1843) -> (-10.099, 5.591)
  line L115 (-9.999, 3.3572) -> (-9.1855, 5.1843)
  line L116 (-10.099, 5.591) -> (-10.9125, 3.7639)
  line L117 (-10.9125, 3.7639) -> (-9.999, 3.3572)
  line L118 (-10.0626, 3.1612) -> (-11.0408, 3.3691)
  line L119 (-10.4785, 1.2049) -> (-10.0626, 3.1612)
  line L120 (-11.0408, 3.3691) -> (-11.4566, 1.4128)
  line L121 (-11.4566, 1.4128) -> (-10.4785, 1.2049)
  point P0 (-11, 0)
  dimension "d47" = 22
  dimension "d48" = 1
  dimension "d49" = 2
  dimension "d52" = 360
  constraints: 244 end point, 2 midpoint, 2 parallel, 1 coincident, 1 horizontal, 1 horizontal alignment, 1 perpendicular, 243 other
  measures "d48" distance of L2.end L1.end
  measures "d49" distance of L1.end L0.end
extrude "擠出8" add sketch "草圖8" along normal blind 1 contours A0 L62 L63 L65 | A0 L65 L64 L62 | L66 L67 L69 A0 | A0 L69 L68 L66 | L61 L60 L58 A0 | A0 L58 L59 L61 | L70 L71 L73 A0 | A0 L73 L72 L70 | L57 L56 L54 A0 | A0 L54 L55 L57 | L74 L75 L77 A0 | A0 L77 L76 L74 | L53 L52 L50 A0 | A0 L50 L51 L53 | L78 L79 L81 A0 | A0 L81 L80 L78 | L49 L48 L46 A0 | A0 L46 L47 L49 | L82 L83 L85 A0 | A0 L85 L84 L82 | L45 L44 L42 A0 | A0 L42 L43 L45 | L86 L87 L89 A0 | A0 L89 L88 L86 | L41 L40 L38 A0 | A0 L38 L39 L41 | L90 L91 L93 A0 | A0 L93 L92 L90 | L37 L36 L34 A0 | A0 L34 L35 L37 | L94 L95 L97 A0 | A0 L97 L96 L94 | L33 L32 L30 A0 | A0 L30 L31 L33 | L98 L99 L101 A0 | A0 L101 L100 L98 | L29 L28 L26 A0 | A0 L26 L27 L29 | L102 L103 L105 A0 | A0 L105 L104 L102 | L25 L24 L22 A0 | A0 L22 L23 L25 | L106 L107 L109 A0 | A0 L109 L108 L106 | L21 L20 L18 A0 | A0 L18 L19 L21 | L110 L111 L113 A0 | A0 L113 L112 L110 | L17 L16 L14 A0 | A0 L14 L15 L17 | L114 L115 L117 A0 | A0 L117 L116 L114 | L13 L12 L10 A0 | A0 L10 L11 L13 | L118 L119 L121 A0 | A0 L121 L120 L118 | L9 L8 L6 A0 | A0 L6 L7 L9 | L2 L1 L0 A0 | A0 L0 L3 L2
sketch "草圖9" plane through (0, -5, 0) normal (0, -1, 0) x (1, 0, 0)
  circle A0 centre (0, 0) radius 11
  line L0 (-1, 10.5) -> (1, 10.5)
  line L1 (1, 10.5) -> (1, 11.5)
  line L2 (1, 11.5) -> (-1, 11.5)
  line L3 (-1, 11.5) -> (-1, 10.5)
  line L4 (-1, 10.5) -> (1, 11.5) construction
  line L5 (1, 10.5) -> (-1, 11.5) construction
  line L6 (-1.4128, 11.4566) -> (-3.3691, 11.0408)
  line L7 (-3.3691, 11.0408) -> (-3.1612, 10.0626)
  line L8 (-3.1612, 10.0626) -> (-1.2049, 10.4785)
  line L9 (-1.2049, 10.4785) -> (-1.4128, 11.4566)
  line L10 (-3.7639, 10.9125) -> (-5.591, 10.099)
  line L11 (-5.591, 10.099) -> (-5.1843, 9.1855)
  line L12 (-5.1843, 9.1855) -> (-3.3572, 9.999)
  line L13 (-3.3572, 9.999) -> (-3.7639, 10.9125)
  line L14 (-5.9505, 9.8915) -> (-7.5685, 8.7159)
  line L15 (-7.5685, 8.7159) -> (-6.9808, 7.9069)
  line L16 (-6.9808, 7.9069) -> (-5.3627, 9.0825)
  line L17 (-5.3627, 9.0825) -> (-5.9505, 9.8915)
  line L18 (-7.877, 8.4381) -> (-9.2153, 6.9519)
  line L19 (-9.2153, 6.9519) -> (-8.4722, 6.2827)
  line L20 (-8.4722, 6.2827) -> (-7.1339, 7.769)
  line L21 (-7.1339, 7.769) -> (-7.877, 8.4381)
  line L22 (-9.4593, 6.616) -> (-10.4593, 4.884)
  line L23 (-10.4593, 4.884) -> (-9.5933, 4.384)
  line L24 (-9.5933, 4.384) -> (-8.5933, 6.116)
  line L25 (-8.5933, 6.116) -> (-9.4593, 6.616)
  line L26 (-10.6281, 4.5048) -> (-11.2462, 2.6026)
  line L27 (-11.2462, 2.6026) -> (-10.2951, 2.2936)
  line L28 (-10.2951, 2.2936) -> (-9.6771, 4.1957)
  line L29 (-9.6771, 4.1957) -> (-10.6281, 4.5048)
  line L30 (-11.3325, 2.1966) -> (-11.5415, 0.2076)
  line L31 (-11.5415, 0.2076) -> (-10.547, 0.103)
  line L32 (-10.547, 0.103) -> (-10.338, 2.0921)
  line L33 (-10.338, 2.0921) -> (-11.3325, 2.1966)
  line L34 (-11.5415, -0.2076) -> (-11.3325, -2.1966)
  line L35 (-11.3325, -2.1966) -> (-10.338, -2.0921)
  line L36 (-10.338, -2.0921) -> (-10.547, -0.103)
  line L37 (-10.547, -0.103) -> (-11.5415, -0.2076)
  line L38 (-11.2462, -2.6026) -> (-10.6281, -4.5048)
  line L39 (-10.6281, -4.5048) -> (-9.6771, -4.1957)
  line L40 (-9.6771, -4.1957) -> (-10.2951, -2.2936)
  line L41 (-10.2951, -2.2936) -> (-11.2462, -2.6026)
  line L42 (-10.4593, -4.884) -> (-9.4593, -6.616)
  line L43 (-9.4593, -6.616) -> (-8.5933, -6.116)
  line L44 (-8.5933, -6.116) -> (-9.5933, -4.384)
  line L45 (-9.5933, -4.384) -> (-10.4593, -4.884)
  line L46 (-9.2153, -6.9519) -> (-7.877, -8.4381)
  line L47 (-7.877, -8.4381) -> (-7.1339, -7.769)
  line L48 (-7.1339, -7.769) -> (-8.4722, -6.2827)
  line L49 (-8.4722, -6.2827) -> (-9.2153, -6.9519)
  line L50 (-7.5685, -8.7159) -> (-5.9505, -9.8915)
  line L51 (-5.9505, -9.8915) -> (-5.3627, -9.0825)
  line L52 (-5.3627, -9.0825) -> (-6.9808, -7.9069)
  line L53 (-6.9808, -7.9069) -> (-7.5685, -8.7159)
  line L54 (-5.591, -10.099) -> (-3.7639, -10.9125)
  line L55 (-3.7639, -10.9125) -> (-3.3572, -9.999)
  line L56 (-3.3572, -9.999) -> (-5.1843, -9.1855)
  line L57 (-5.1843, -9.1855) -> (-5.591, -10.099)
  line L58 (-3.3691, -11.0408) -> (-1.4128, -11.4566)
  line L59 (-1.4128, -11.4566) -> (-1.2049, -10.4785)
  line L60 (-1.2049, -10.4785) -> (-3.1612, -10.0626)
  line L61 (-3.1612, -10.0626) -> (-3.3691, -11.0408)
  line L62 (-1, -11.5) -> (1, -11.5)
  line L63 (1, -11.5) -> (1, -10.5)
  line L64 (1, -10.5) -> (-1, -10.5)
  line L65 (-1, -10.5) -> (-1, -11.5)
  line L66 (1.4128, -11.4566) -> (3.3691, -11.0408)
  line L67 (3.3691, -11.0408) -> (3.1612, -10.0626)
  line L68 (3.1612, -10.0626) -> (1.2049, -10.4785)
  line L69 (1.2049, -10.4785) -> (1.4128, -11.4566)
  line L70 (3.7639, -10.9125) -> (5.591, -10.099)
  line L71 (5.591, -10.099) -> (5.1843, -9.1855)
  line L72 (5.1843, -9.1855) -> (3.3572, -9.999)
  line L73 (3.3572, -9.999) -> (3.7639, -10.9125)
  line L74 (5.9505, -9.8915) -> (7.5685, -8.7159)
  line L75 (7.5685, -8.7159) -> (6.9808, -7.9069)
  line L76 (6.9808, -7.9069) -> (5.3627, -9.0825)
  line L77 (5.3627, -9.0825) -> (5.9505, -9.8915)
  line L78 (7.877, -8.4381) -> (9.2153, -6.9519)
  line L79 (9.2153, -6.9519) -> (8.4722, -6.2827)
  line L80 (8.4722, -6.2827) -> (7.1339, -7.769)
  line L81 (7.1339, -7.769) -> (7.877, -8.4381)
  line L82 (9.4593, -6.616) -> (10.4593, -4.884)
  line L83 (10.4593, -4.884) -> (9.5933, -4.384)
  line L84 (9.5933, -4.384) -> (8.5933, -6.116)
  line L85 (8.5933, -6.116) -> (9.4593, -6.616)
  line L86 (10.6281, -4.5048) -> (11.2462, -2.6026)
  line L87 (11.2462, -2.6026) -> (10.2951, -2.2936)
  line L88 (10.2951, -2.2936) -> (9.6771, -4.1957)
  line L89 (9.6771, -4.1957) -> (10.6281, -4.5048)
  line L90 (11.3325, -2.1966) -> (11.5415, -0.2076)
  line L91 (11.5415, -0.2076) -> (10.547, -0.103)
  line L92 (10.547, -0.103) -> (10.338, -2.0921)
  line L93 (10.338, -2.0921) -> (11.3325, -2.1966)
  line L94 (11.5415, 0.2076) -> (11.3325, 2.1966)
  line L95 (11.3325, 2.1966) -> (10.338, 2.0921)
  line L96 (10.338, 2.0921) -> (10.547, 0.103)
  line L97 (10.547, 0.103) -> (11.5415, 0.2076)
  line L98 (11.2462, 2.6026) -> (10.6281, 4.5048)
  line L99 (10.6281, 4.5048) -> (9.6771, 4.1957)
  line L100 (9.6771, 4.1957) -> (10.2951, 2.2936)
  line L101 (10.2951, 2.2936) -> (11.2462, 2.6026)
  line L102 (10.4593, 4.884) -> (9.4593, 6.616)
  line L103 (9.4593, 6.616) -> (8.5933, 6.116)
  line L104 (8.5933, 6.116) -> (9.5933, 4.384)
  line L105 (9.5933, 4.384) -> (10.4593, 4.884)
  line L106 (9.2153, 6.9519) -> (7.877, 8.4381)
  line L107 (7.877, 8.4381) -> (7.1339, 7.769)
  line L108 (7.1339, 7.769) -> (8.4722, 6.2827)
  line L109 (8.4722, 6.2827) -> (9.2153, 6.9519)
  line L110 (7.5685, 8.7159) -> (5.9505, 9.8915)
  line L111 (5.9505, 9.8915) -> (5.3627, 9.0825)
  line L112 (5.3627, 9.0825) -> (6.9808, 7.9069)
  line L113 (6.9808, 7.9069) -> (7.5685, 8.7159)
  line L114 (5.591, 10.099) -> (3.7639, 10.9125)
  line L115 (3.7639, 10.9125) -> (3.3572, 9.999)
  line L116 (3.3572, 9.999) -> (5.1843, 9.1855)
  line L117 (5.1843, 9.1855) -> (5.591, 10.099)
  line L118 (3.3691, 11.0408) -> (1.4128, 11.4566)
  line L119 (1.4128, 11.4566) -> (1.2049, 10.4785)
  line L120 (1.2049, 10.4785) -> (3.1612, 10.0626)
  line L121 (3.1612, 10.0626) -> (3.3691, 11.0408)
  point P0 (0, 11)
  dimension "d56" = 22
  dimension "d57" = 2
  dimension "d58" = 1
  dimension "d61" = 360
  constraints: 244 end point, 2 midpoint, 2 parallel, 1 coincident, 1 horizontal, 1 perpendicular, 1 vertical alignment, 243 other
  measures "d57" distance of L2.end L1.end
  measures "d58" distance of L1.end L0.end
extrude "擠出9" add sketch "草圖9" along normal blind 1 contours L97 L96 L95 A0 | A0 L95 L94 L97 | L91 L90 L93 A0 | A0 L93 L92 L91 | L101 L100 L99 A0 | A0 L99 L98 L101 | L87 L86 L89 A0 | A0 L89 L88 L87 | L105 L104 L103 A0 | A0 L103 L102 L105 | L83 L82 L85 A0 | A0 L85 L84 L83 | L109 L108 L107 A0 | A0 L107 L106 L109 | L79 L78 L81 A0 | A0 L81 L80 L79 | L113 L112 L111 A0 | A0 L111 L110 L113 | L75 L74 L77 A0 | A0 L77 L76 L75 | L117 L116 L115 A0 | A0 L115 L114 L117 | L71 L70 L73 A0 | A0 L73 L72 L71 | L121 L120 L119 A0 | A0 L119 L118 L121 | L67 L66 L69 A0 | A0 L69 L68 L67 | L1 L0 L3 A0 | A0 L3 L2 L1 | L63 L62 L65 A0 | A0 L65 L64 L63 | L9 L8 L7 A0 | A0 L7 L6 L9 | L59 L58 L61 A0 | A0 L61 L60 L59 | L13 L12 L11 A0 | A0 L11 L10 L13 | L55 L54 L57 A0 | A0 L57 L56 L55 | L17 L16 L15 A0 | A0 L15 L14 L17 | L51 L50 L53 A0 | A0 L53 L52 L51 | L21 L20 L19 A0 | A0 L19 L18 L21 | L47 L46 L49 A0 | A0 L49 L48 L47 | L25 L24 L23 A0 | A0 L23 L22 L25 | L43 L42 L45 A0 | A0 L45 L44 L43 | L29 L28 L27 A0 | A0 L27 L26 L29 | L39 L38 L41 A0 | A0 L41 L40 L39 | L33 L32 L31 A0 | A0 L31 L30 L33 | L35 L34 L37 A0 | A0 L37 L36 L35